Haken_Kleiderschrank_v1 (Autodesk Fusion 360 design; units mm, degrees)
Autodesk Fusion 360 part; units mm, degrees
note: some values were not read from the file. Set by a fixed rule: which sketch regions a step uses.
sketch "Skizze1" plane through (0, 0, 0) normal (0, 1, 0) x (1, 0, 0)
  line L0 (-10, -11) -> (10, -11)
  arc A0 (10, -11) -> (10, 11) centre (10, 0) ccw
  line L1 (10, 11) -> (-10, 11)
  arc A1 (-10, 11) -> (-10, -11) centre (-10, 0) ccw
  line L2 (-10, 0) -> (10, 0) construction
  line L3 (0, 0) -> (16, 0)
  line L4 (0, 0) -> (-16, 0)
  circle A2 centre (-16, 0) radius 2.4
  circle A3 centre (16, 0) radius 2.4
  line L5 (21, 0) -> (4.3, 0)
  circle A4 centre (4.3, 0) radius 2
  line L6 (21, 0) -> (-13, 0)
  circle A5 centre (-2, 0) radius 11
  circle A6 centre (-2, 0) radius 7.55
  line L7 (-2, 7.55) -> (10, 7.55)
  line L8 (-2, -7.55) -> (10, -7.55)
  circle A7 centre (10, -9.275) radius 1.725
  circle A8 centre (10, 9.275) radius 1.725
  dimension "d1" = 22
  dimension "d2" = 16
  dimension "d3" = 16
  dimension "d4" = 4.8
  dimension "d5" = 4.8
  dimension "d6" = 16.7
  dimension "d7" = 4
  dimension "d8" = 34
  dimension "d9" = 15.1
  constraint tangent L0 A0
  constraint tangent A0 L1
  constraint parallel L0 L1
  constraint tangent L1 A1
  constraint tangent L0 A1
  constraint horizontal L2
  constraint coincident L3.start L4.start
  constraint midpoint L2 L3.start
  constraint parallel L2 L3
  constraint parallel L2 L4
  constraint coincident L4.end A2.centre
  constraint coincident L3.end A3.centre
  constraint midpoint A0 L5.start
  constraint parallel L3 L5
  constraint coincident L5.end A4.centre
  constraint parallel L2 L6
  constraint coincident L6.end A5
  constraint concentric A5 A6
  constraint coincident A6 L7.start
  constraint tangent A6 L7
  constraint parallel L4 L7
  constraint coincident A6 L8.start
  constraint tangent A6 L8
  constraint parallel L2 L8
  constraint coincident L0.end A7
  constraint coincident L8.end A7
  constraint coincident L7.end A8
  constraint coincident A0.end A8
  measures "d1" diameter of A0
  measures "d2" distance of L3.start L3.end
  measures "d3" distance of L3.start L4.end
  measures "d4" diameter of A2
  measures "d5" diameter of A3
  measures "d6" distance of L5.start L5.end
  measures "d7" diameter of A4
  measures "d8" distance of L5.start L6.end
  measures "d9" diameter of A6
extrude "Extrusion1" add sketch "Skizze1" along normal blind 2.9 contours L0 L1 A1 A5 | L0 A5 L8 A7 | L4 L6 A5 A6 L8 | A0 L3 A3 L5 L6 A5 L8 A7 | A7 | L4 L6 A5 A6 L7 | L3 L5 A4 L6 A5 A6 L8 | L1 A5 L7 A8 | A0 L3 A3 L5 L6 A5 L7 A8 | L3 L4 A4 L6 A6 | L3 L4 A4 L6 A6 | L3 L5 A4 L6 A5 A6 L7 | A8 | L3 A3 L5 L6 | L3 A3 L5 L6 | A2 makes body 1
extrude "Extrusion2" add sketch "Skizze1" against normal blind 7.1 contours L3 A3 L5 L6 | L3 A3 L5 L6 | A2 bodies 1
extrude "Extrusion3" add sketch "Skizze1" along normal blind 2.9 separate body contours L0 A5 L8 A7 | L4 L6 A5 A6 L8 | A7 | L4 L6 A5 A6 L7 | L1 A5 L7 A8 | A8 makes body 2
sketch "Skizze2" plane through (0, 2.9, 0) normal (0, 1, 0) x (-1, 0, 0)
  line L0 (2, -7.55) -> (-10, -7.55)
  arc A0 (-10, -7.55) -> (-10, -11) centre (-10, -9.275) ccw
  line L1 (-10, -11) -> (2.0007, -11)
  arc A1 (2.0007, -11) -> (2.0007, 11) centre (2, 0) ccw
  line L2 (2.0007, 11) -> (-10, 11)
  arc A2 (-10, 11) -> (-10, 7.55) centre (-10, 9.275) ccw
  line L3 (-10, 7.55) -> (2, 7.55)
  arc A3 (2, -7.55) -> (2, 7.55) centre (2, 0) ccw
extrude "Extrusion4" add sketch "Skizze2" along normal blind 11.8 separate body makes body 3
sketch "Skizze3" plane through (0, 14.7, 0) normal (0, 1, 0) x (-1, 0, 0)
  line L0 (-10, -11) -> (2.0007, -11)
  arc A0 (2.0007, -11) -> (2.0007, 11) centre (2, 0) ccw
  line L1 (2.0007, 11) -> (-10, 11)
  arc A1 (2, -7.55) -> (2, 7.55) centre (2, 0) ccw
  line L2 (-10, 0) -> (-10, 6.45)
  line L3 (-10, -6.45) -> (-10, 0)
  line L4 (2, -7.55) -> (-10, -6.45)
  line L5 (2, 7.55) -> (-10, 6.45)
  arc A2 (-9.5864, -6.4879) -> (-10, -11) centre (-10, -8.725) ccw
  arc A3 (-10, 11) -> (-9.5864, 6.4879) centre (-10, 8.725) ccw
  dimension "d20" = 6.45
  dimension "d21" = 6.45
  constraint coincident A1.start L4.start
  constraint coincident A1.end L5.start
  constraint coincident L2.end A3
  constraint coincident L3.start A2
  constraint coincident L4 A2.start
  constraint coincident L5 A3.end
  measures "d20" distance of L2.start L2.end
  measures "d21" distance of L3.start L2.start
loft "Erhebung1" add profiles "Skizze3" section 1 face at (4.6666, 2.9, 9.85) section 2 contours L0 A0 L1 A1 L4 L5 A2 A3 separate body on bodies 2 makes body 4
chamfer "Fase1" distance 2.5 angle 45 1 edges at (2.4353, 2.9, -0.7232) on bodies 1
fillet "Abrundung1" radius 0.3 8 edges at (-9.55, 14.7, 0) (4, 14.7, 7) (12.275, 14.7, 8.725) (3.9996, 14.7, 11) (-13, 14.7, 0) (3.9996, 14.7, -11) (12.275, 14.7, -8.725) (4, 14.7, -7) on bodies 4
fillet "Abrundung2" radius 0.4 2 edges at (-18.2376, -7.1, -0.8679) (13.7624, -7.1, -0.8679) on bodies 1
